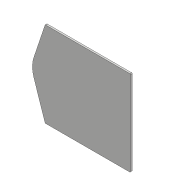
# Autodesk Inventor part: RPi_mount
Saved by Autodesk Inventor 2018 (Build 220112000, 112)
## iProperties
Created: 2019-11-28
Part Number: RPi_mount
Material: Generic
Document SubType Name: Modeling
Designer: Clevo
Density: 1 g/cm^3
Appearance: Default
Author: Clevo
Autodesk Inventor part; units mm, degrees
ref_plane "YZ Plane" through (0, 0, 0) normal (1, 0, 0) x (0, 1, 0)
ref_plane "XZ Plane" through (0, 0, 0) normal (0, 1, 0) x (-1, 0, 0)
ref_plane "XY Plane" through (0, 0, 0) normal (0, 0, 1) x (1, 0, 0)
sketch "Sketch1" plane through (0, 0, 0) normal (0, 1, 0) x (-1, 0, 0)
  circle A0 centre (0, 0) radius 50
  line L0 (47.697, 15) -> (-47.697, 15)
  line L1 (-47.697, 15) -> (-47.697, -15)
  line L2 (-47.697, -15) -> (47.697, -15)
  line L3 (47.697, -15) -> (47.697, 15)
  line L4 (47.697, 15) -> (27.697, 15)
  line L5 (27.697, 15) -> (27.697, -15)
  line L6 (27.697, -15) -> (47.697, -15)
  line L7 (47.697, -15) -> (47.697, 15)
  dimension "d0" = 100
  dimension "d1" = 30
  dimension "d22" = 20
  constraints: 16 end point, 4 parallel, 3 point on circle, 2 horizontal, 2 perpendicular, 1 centre point, 1 coincident
  measures "d0" diameter of A0
  measures "d1" distance of L2.end L0.start
  measures "d22" distance between parallel lines of L3 L5
extrude "Extrusion1" add sketch "Sketch1" along normal blind 30 contours A0 L3 | L3 L2 L5 L0
sketch "Sketch2" plane through (0, 0, 0) normal (0, -1, 0) x (1, 0, 0)
  line L0 (122.303, 75) -> (-27.697, 75)
  line L1 (-27.697, 75) -> (-27.697, -75)
  line L2 (-27.697, -75) -> (122.303, -75)
  line L3 (122.303, -75) -> (122.303, 75)
  line L4 (-27.697, 15) -> (-27.697, -15) projected
  arc A0 (-47.697, 15) -> (-47.697, -15) centre (0, 0) ccw projected
  line L5 (-27.697, -15) -> (-47.697, -15) projected
  line L6 (-27.697, 15) -> (-27.697, -15) projected
  line L7 (-47.697, 15) -> (-27.697, 15) projected
  line L8 (-27.697, -75) -> (-47.697, -15)
  line L9 (-47.697, 15) -> (-27.697, 15) projected
  line L10 (-27.697, 75) -> (-47.697, 15)
  point P0 (-27.697, 0)
  dimension "d4" = 150
  dimension "d5" = 150
  constraints: 12 end point, 2 parallel, 1 horizontal, 1 midpoint, 1 perpendicular, 2 other
  measures "d4" distance of L1.end L2.end
  measures "d5" distance of L2.end L0.start
extrude "Extrusion2" add sketch "Sketch2" against normal blind 3 contours L3 L2 L1 L0 | L1 L7 L10 | L8 L5 L1
sketch "Sketch3" plane through (0, 3, 0) normal (0, 1, 0) x (1, 0, 0)
  arc A0 (-47.697, 15) -> (-47.697, -15) centre (0, 0) ccw projected
  line L0 (-47.697, -15) -> (-27.697, -15) projected
  line L1 (-27.697, -15) -> (-27.697, 15) projected
  line L2 (-27.697, 15) -> (-47.697, 15) projected
  line L3 (-27.697, 15) -> (12.303, 15)
  line L4 (12.303, 15) -> (12.303, -15)
  line L5 (12.303, -15) -> (-27.697, -15)
  line L6 (-27.697, -15) -> (-27.697, 15)
  line L7 (-47.697, -15) -> (-27.697, -15) projected
  dimension "d8" = 40
  constraints: 8 end point, 2 parallel, 1 collinear, 1 horizontal, 1 perpendicular
  measures "d8" distance of L4.end L5.end
extrude "Extrusion3" add sketch "Sketch3" along normal blind 15 contours L3 L4 L5 L1
sketch "Sketch4" plane through (0, 18, 0) normal (0, 1, 0) x (1, 0, 0)
  line L0 (-27.697, -15) -> (-27.697, 15) projected
  line L1 (-27.697, -15) -> (12.303, -15) projected
  line L2 (12.303, -15) -> (12.303, 15) projected
  line L3 (12.303, 15) -> (-27.697, 15) projected
  line L4 (4.303, -2.5) -> (-16.697, -2.5)
  line L5 (-16.697, -2.5) -> (-16.697, 10)
  line L6 (-16.697, 10) -> (4.303, 10)
  line L7 (4.303, 10) -> (4.303, -2.5)
  circle A0 centre (4.303, -2.5) radius 2.5
  circle A1 centre (-16.697, -2.5) radius 2.5
  circle A2 centre (4.303, 10) radius 2.5
  circle A3 centre (-16.697, 10) radius 2.5
  point P0 (0, 0)
  dimension "d11" = 12.5
  dimension "d12" = 21
  dimension "d13" = 8
  dimension "d14" = 5
  dimension "d15" = 5
  dimension "d16" = 5
  dimension "d17" = 5
  dimension "d18" = 5
  constraints: 8 end point, 4 centre point, 4 coincident, 2 parallel, 1 horizontal, 1 perpendicular
  measures "d11" distance of L6.end L4.start
  measures "d12" distance of L4.start L4.end
  measures "d13" distance between parallel lines of L2 L7
  measures "d14" distance between parallel lines of L3 L6
  measures "d15" diameter of A0
  measures "d16" diameter of A1
  measures "d17" diameter of A3
  measures "d18" diameter of A2
extrude "Extrusion4" add sketch "Sketch4" along normal blind 7 contours A1 L5 L4 | L4 L5 A1 | A0 L7 L4 | L4 L7 A0 | A3 L6 L5 | L5 L6 A3 | A2 L6 L7 | L7 L6 A2
fillet "Fillet1" radius 2 4 edges at (1.803, 18, -10) (-19.197, 18, -10) (-19.197, 18, 2.5) (1.803, 18, 2.5)
sketch "Sketch5" plane through (12.303, 3, 15) normal (1, 0, 0) x (0, 0, -1)
  line L0 (30, 0) -> (0, 0) projected
  line L1 (30, 0) -> (30, 15) projected
  line L2 (0, 15) -> (30, 15) projected
  line L3 (0, 0) -> (0, 15) projected
  point P0 (15, -3)
  point P1 (15, 7.5)
  point P2 (0, 7.5)
  point P3 (15, 15)
  constraints: 2 midpoint, 1 horizontal alignment, 1 vertical alignment
hole "Hole1" at (12.303, 10.5, 0) direction (-1, 0, 0) diameter 4.5 end through all counterbore diameter 8 counterbore depth 55 clearance for "Socket Head Cap Screw" size "M4" standard "Ansi Metric M Profile"
fillet "Fillet2" radius 1 1 edges at (12.303, 10.5, 4)
sketch "Sketch6" plane through (4.303, 25, 2.5) normal (0, 1, 0) x (1, 0, 0)
  circle A0 centre (0, 0) radius 2.5 projected
  circle A1 centre (-21, 0) radius 2.5 projected
  circle A2 centre (-21, 12.5) radius 2.5 projected
  circle A3 centre (0, 12.5) radius 2.5 projected
  point P0 (-4.303, 2.5)
hole "Hole2" at (4.303, 25, 2.5) at (-16.697, 25, 2.5) at (-16.697, 25, -10) at (4.303, 25, -10) direction (0, -1, 0) diameter 1.567 depth 10 tip angle 118 thread size "M2x0.4" class "6H" standard "ANSI Metric M Profile"
fillet "Fillet3" radius 1 13 edges at (122.303, 1.5, -75) (-27.697, 1.5, -75) (122.303, 1.5, 75) (-27.697, 1.5, 75) (-17.697, 3, 15) (-47.697, 16.5, 15) (-17.697, 3, -15) (-47.697, 16.5, -15) (-27.697, 18, 0) (-27.697, 30, 0) (12.303, 3, 0) (12.303, 10.5, -15) (12.303, 10.5, 15)
equation "\"d15\" = d16"
equation "\"d17\" = d16"
equation "\"d18\" = d17"
body "Solid1"
